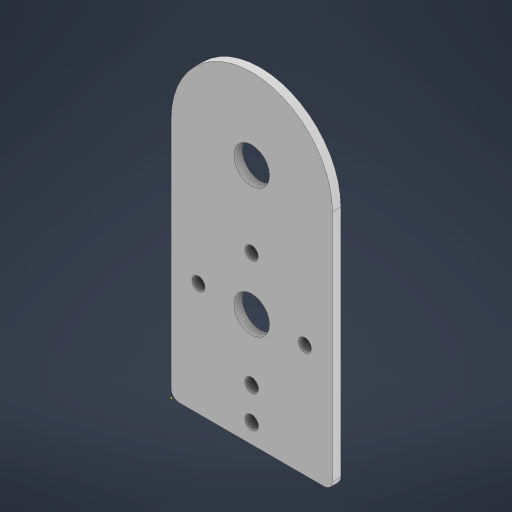
# Autodesk Inventor part: wrist plate 2
Saved by Autodesk Inventor 2024 (Build 280153000, 153)
## iProperties
Created: 2023-11-09
Part Number: wrist plate 2
Material: Generic
Document SubType Name: Modeling
Designer: ellen
Density: 1 g/cm^3
Appearance: Default
Author: ellen
Autodesk Inventor part; units mm, degrees
ref_plane "YZ Plane" through (0, 0, 0) normal (1, 0, 0) x (0, 1, 0)
ref_plane "XZ Plane" through (0, 0, 0) normal (0, 1, 0) x (-1, 0, 0)
ref_plane "XY Plane" through (0, 0, 0) normal (0, 0, 1) x (1, 0, 0)
sketch "Sketch1" plane through (0, 0, 0) normal (0, 0, 1) x (1, 0, 0)
  line L0 (0, 0) -> (63.5, 0)
  line L1 (63.5, 0) -> (63.5, 127)
  line L2 (63.5, 127) -> (0, 127)
  line L3 (0, 127) -> (0, 0)
  circle A0 centre (31.75, 95.25) radius 7
  circle A1 centre (31.75, 44.45) radius 7
  circle A2 centre (31.75, 20.32) radius 2.6543
  circle A3 centre (31.75, 7.62) radius 2.6543
  dimension "d0" = 63.5
  dimension "d1" = 127
  dimension "d2" = 119.38
  dimension "d3" = 106.68
  dimension "d4" = 31.75
  dimension "d5" = 82.55
  dimension "d12" = 14
  dimension "d13" = 14
  dimension "d14" = 5.3086
  dimension "d15" = 5.3086
  constraints: 8 end point, 4 centre point, 2 parallel, 1 horizontal, 1 perpendicular
  measures "d0" distance of L2.end L1.end
  measures "d1" distance of L1.end L0.end
  measures "d2" distance from line of L2 A3.centre
  measures "d3" distance from line of L2 A2.centre
  measures "d4" distance from line of L2 A0.centre
  measures "d5" distance from line of L2 A1.centre
  measures "d12" diameter of A0
  measures "d13" diameter of A1
  measures "d14" diameter of A2
  measures "d15" diameter of A3
extrude "Extrusion1" add sketch "Sketch1" along normal blind 3.302
fillet "Fillet1" radius 31.75 1 edges at (63.5, 127, 1.651)
fillet "Fillet2" radius 31.75 1 edges at (0, 127, 1.651)
fillet "Fillet3" radius 3.175 1 edges at (63.5, 0, 1.651)
fillet "Fillet4" radius 3.175 1 edges at (0, 0, 1.651)
sketch "Sketch2" plane through (0, 0, 3.302) normal (0, 0, 1) x (1, 0, 0)
  point P0 (0, 0)
sketch "Sketch3" plane through (0, 0, 3.302) normal (0, 0, 1) x (1, 0, 0)
  circle A0 centre (31.75, 44.45) radius 7 projected
  circle A1 centre (31.75, 44.45) radius 20.955
  line L0 (31.75, 44.45) -> (31.75, 96.3454)
  line L1 (31.75, 44.45) -> (1.7281, 44.45)
  line L2 (31.75, 44.45) -> (60.8223, 44.45)
  point P0 (0, 0)
  point P1 (31.75, 65.405)
  point P2 (52.705, 44.45)
  point P3 (10.795, 44.45)
  dimension "d16" = 41.91
  constraints: 6 end point, 3 point on circle, 3 point on line, 2 horizontal, 1 centre point, 1 coincident, 1 vertical
  measures "d16" diameter of A1
hole "Hole1" at (31.75, 65.405, 3.302) at (52.705, 44.45, 3.302) at (10.795, 44.45, 3.302) direction (0, 0, -1) diameter 5.1054 depth 16.256 tip angle 118 clearance for "Flat Head Machine Screw (82)" size "#10" standard "Ansi Unified Screw Threads"
body "Solid1"
